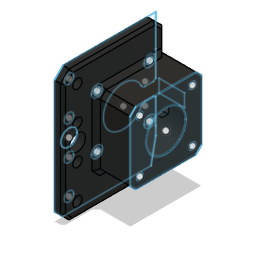
X Axis motor mount (Autodesk Fusion 360 design; units mm, degrees)
Autodesk Fusion 360 part; units mm, degrees
sketch "sketch 905" plane through (736, 0, 0) normal (-1, 0, 0) x (0, 0, 1)
  circle A0 centre (-248.0507, 157.3963) radius 1.75
  circle A1 centre (-263.5507, 141.8963) radius 11.75
  circle A2 centre (-279.0507, 126.3963) radius 1.75
  circle A3 centre (-279.0507, 157.3963) radius 1.75
  circle A4 centre (-248.0507, 126.3963) radius 1.75
  line L0 (-245.8007, 162.8963) -> (-281.3007, 162.8963)
  line L1 (-281.3007, 162.8963) -> (-284.5507, 159.6463)
  line L2 (-284.5507, 159.6463) -> (-284.5507, 124.1463)
  line L3 (-284.5507, 124.1463) -> (-281.3007, 120.8963)
  line L4 (-281.3007, 120.8963) -> (-245.8007, 120.8963)
  line L5 (-245.8007, 120.8963) -> (-242.5507, 124.1463)
  line L6 (-242.5507, 124.1463) -> (-242.5507, 159.6463)
  line L7 (-242.5507, 159.6463) -> (-245.8007, 162.8963)
extrude "Extrude1" add sketch "sketch 905" along normal blind 25
chamfer "Chamfer1" distance 1.9 angle 45 1 edges at (711, 141.8963, -284.5507)
sketch "sketch 954" plane through (0, 0, -284.5507) normal (0, 0, -1) x (-1, 0, 0)
  line L0 (-711, 138.1463) -> (-726, 138.1463)
  line L1 (-711, 145.6463) -> (-711, 138.1463)
  line L2 (-726, 145.6463) -> (-711, 145.6463)
  line L3 (-726, 138.1463) -> (-726, 145.6463)
extrude "Extrude2" cut sketch "sketch 954" against normal blind 21
chamfer "Chamfer2" distance 1.5 angle 45 2 edges at (726, 145.6463, -279.6185) (726, 138.1463, -279.6185)
chamfer "Chamfer3" distance 1 angle 45 7 edges at (718.7, 145.6463, -284.5507) (725.25, 144.8963, -284.5507) (726, 141.8963, -284.5507) (725.25, 138.8963, -284.5507) (718.7, 138.1463, -284.5507) (711.95, 138.1463, -283.6007) (711.95, 145.6463, -283.6007)
fillet "Fillet1" radius 2.5 2 edges at (717.75, 138.1463, -274.6862) (717.75, 145.6463, -274.6862)
sketch "sketch 975" plane through (711, 0, 0) normal (-1, 0, 0) x (0, 0, 1)
  circle A0 centre (-231.5507, 171.8963) radius 2.75
  circle A1 centre (-231.5507, 131.8963) radius 2.75
  circle A2 centre (-231.5507, 141.8963) radius 4.75
  circle A3 centre (-231.5507, 141.8963) radius 4.75
  circle A4 centre (-231.5507, 111.8963) radius 2.75
  circle A5 centre (-279.0507, 126.3963) radius 1.75
  circle A6 centre (-248.0507, 126.3963) radius 1.75
  circle A7 centre (-279.0507, 157.3963) radius 1.75
  circle A8 centre (-231.5507, 151.8963) radius 2.75
  circle A9 centre (-248.0507, 157.3963) radius 1.75
  line L0 (-223.0507, 175.3963) -> (-228.0507, 180.3963)
  line L1 (-228.0507, 180.3963) -> (-282.6507, 180.3963)
  line L2 (-282.6507, 180.3963) -> (-282.6507, 161.5463)
  line L3 (-282.6507, 161.5463) -> (-282.6507, 146.6463)
  line L4 (-282.6507, 146.6463) -> (-281.2365, 145.6463)
  line L5 (-281.2365, 145.6463) -> (-276.3569, 145.6463)
  arc A10 (-276.3569, 145.6463) -> (-274.1102, 147.0499) centre (-276.3569, 148.1463) ccw
  arc A11 (-274.1102, 136.7428) -> (-274.1102, 147.0499) centre (-263.5507, 141.8963) ccw
  arc A12 (-274.1102, 136.7428) -> (-276.3569, 138.1463) centre (-276.3569, 135.6463) ccw
  line L6 (-276.3569, 138.1463) -> (-281.2365, 138.1463)
  line L7 (-281.2365, 138.1463) -> (-282.6507, 137.1463)
  line L8 (-282.6507, 137.1463) -> (-282.6507, 122.2463)
  line L9 (-282.6507, 122.2463) -> (-282.6507, 117.3357)
  line L10 (-282.6507, 122.2463) -> (-282.6507, 117.3357)
  line L11 (-282.6507, 117.3357) -> (-279.8748, 103.3963)
  line L12 (-282.6507, 117.3357) -> (-279.8748, 103.3963)
  line L13 (-228.0507, 103.3963) -> (-279.8748, 103.3963)
  line L14 (-223.0507, 108.3963) -> (-228.0507, 103.3963)
  line L15 (-223.0507, 175.3963) -> (-223.0507, 108.3963)
extrude "Extrude3" add sketch "sketch 975" against normal blind 5
chamfer "Chamfer4" distance 5 angle 45 2 edges at (713.5, 180.3963, -282.6507) (713.5, 103.3963, -279.8748)
chamfer "Chamfer5" distance 1.5 angle 45 10 edges at (716, 168.4713, -282.6507) (716, 177.8963, -280.1507) (716, 180.3963, -252.8507) (716, 177.8963, -225.5507) (716, 141.8963, -223.0507) (716, 105.8963, -225.5507) (716, 103.3963, -251.4627) (716, 105.8482, -277.863) (716, 112.8179, -281.751) (716, 119.791, -282.6507)
chamfer "Chamfer6" distance 2.5 angle 45 5 edges at (716, 162.8963, -263.4757) (716, 161.2713, -244.1757) (716, 141.8963, -242.5507) (716, 122.5213, -244.1757) (716, 120.8963, -263.4757)
sketch "sketch 1076" plane through (711, 0, 0.1093) normal (-1, 0, 0) x (0, 0, 1)
  circle A0 centre (-248.16, 157.3963) radius 1.75
  circle A1 centre (-248.16, 157.3963) radius 3.25
  circle A2 centre (-279.16, 126.3963) radius 1.75
  circle A3 centre (-279.16, 126.3963) radius 3.25
  circle A4 centre (-279.16, 157.3963) radius 1.75
  circle A5 centre (-279.16, 157.3963) radius 3.25
  circle A6 centre (-248.16, 126.3963) radius 1.75
  circle A7 centre (-248.16, 126.3963) radius 3.25
extrude "Extrude4" cut sketch "sketch 1076" against normal blind 12.5
chamfer "Chamfer7" distance 1.5 angle 45 4 edges at (723.5, 158.0292, -277.4191) (723.5, 127.0292, -277.4191) (723.5, 158.0292, -246.4191) (723.5, 127.0292, -246.4191)
